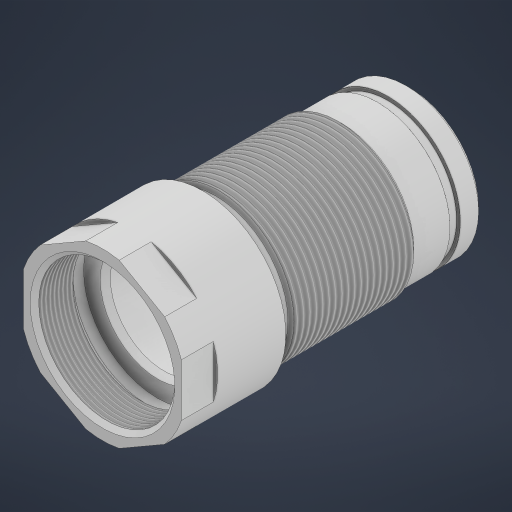
# Autodesk Inventor part: Переводник
Saved by Autodesk Inventor 2024.3 (Build 283343000, 343)
## iProperties
Created: 2025-08-06
Part Number: Переводник
Material: Generic
Document SubType Name: Modeling
Designer: LeoFB
Density: 1 g/cm^3
Appearance: Default
Author: LeoFB
Autodesk Inventor part; units mm, degrees
ref_plane "YZ Plane" through (0, 0, 0) normal (1, 0, 0) x (0, 1, 0)
ref_plane "XZ Plane" through (0, 0, 0) normal (0, 1, 0) x (-1, 0, 0)
ref_plane "XY Plane" through (0, 0, 0) normal (0, 0, 1) x (1, 0, 0)
sketch "Sketch1" plane through (0, 0, 0) normal (0, 1, 0) x (-1, 0, 0)
  line L0 (34, 0) -> (64.4, 0) construction
  line L1 (34, 32) -> (36, 32) construction
  line L2 (34, 91) -> (34, 97)
  line L3 (34, 97) -> (34, 91)
  line L4 (34, 91) -> (35.4142, 89.5858)
  line L5 (35.4142, 89.5858) -> (35.4142, 89.5858)
  line L6 (35.4142, 89.5858) -> (35.4142, 33.4142)
  line L7 (34, 97) -> (39, 97)
  line L8 (34, 97) -> (39, 97) construction
  line L9 (39, 97) -> (39, 129)
  line L10 (39, 129) -> (36, 129)
  line L11 (36, 129) -> (36, 144)
  line L12 (33.9171, 144) -> (36, 144)
  line L13 (31.9171, 142) -> (31.9171, 125.958)
  line L14 (31.9171, 144) -> (47.9592, 144) construction
  line L15 (31.9171, 125.958) -> (34.7455, 123.1296)
  line L16 (31.9171, 125.958) -> (35.9171, 125.958) construction
  line L17 (34.7455, 123.1296) -> (34.7455, 118.1296)
  line L18 (34.7455, 118.1296) -> (26.9171, 118.1296)
  line L19 (26.9171, 118.1296) -> (25.1856, 115.1305)
  line L20 (26.9171, 118.1296) -> (30.3802, 118.1296) construction
  line L21 (25.1856, 42.2286) -> (28.1856, 37.0325)
  line L22 (25.1856, 42.2286) -> (31.1856, 42.2286) construction
  line L23 (28.1856, 37.0325) -> (28.1856, 1.6)
  line L24 (32.4, 0) -> (29.7856, 0)
  line L25 (28.1856, 1.6) -> (29.7856, 0)
  line L26 (34, 1.6) -> (32.4, 0)
  line L27 (33.9171, 144) -> (31.9171, 142)
  line L28 (33.9, 14.92) -> (32.5, 14.92)
  line L29 (32.4, 14.82) -> (32.4, 10.32)
  line L30 (32.5, 10.22) -> (33.9, 10.22)
  line L31 (34, 1.6) -> (34, 10.12)
  arc A0 (32.5, 14.92) -> (32.4, 14.82) centre (32.5, 14.82) ccw
  arc A1 (32.4, 10.32) -> (32.5, 10.22) centre (32.5, 10.32) ccw
  arc A2 (33.9, 14.92) -> (34, 15.02) centre (33.9, 15.02) ccw
  arc A3 (34, 10.12) -> (33.9, 10.22) centre (33.9, 10.12) ccw
  line L32 (34, 15.02) -> (34, 32)
  line L33 (34, 32) -> (35.4142, 33.4142)
  line L34 (25.1856, 115.1305) -> (25.1856, 42.2286)
  line L35 (0, -28.8) -> (0, 172.8001) projected
  point P0 (0, 0)
  point P1 (28.1856, 0)
  point P2 (32.4, 14.92)
  point P3 (32.4, 10.22)
  dimension "d2" = 32
  dimension "d4" = 2
  dimension "d8" = 65
  dimension "d12" = 5
  dimension "d14" = 32
  dimension "d16" = 90
  dimension "d18" = 90
  dimension "d22" = 90
  dimension "d23" = 4
  dimension "d24" = 45
  dimension "d25" = 5
  dimension "d26" = 135
  dimension "d28" = 120
  dimension "d30" = 6
  dimension "d31" = 60
  dimension "d32" = 150
  dimension "d33" = 1.6
  dimension "d34" = 1.6
  dimension "d35" = 1.6
  dimension "d36" = 1.6
  dimension "d37" = 2
  dimension "d38" = 2
  dimension "d39" = 4.7
  dimension "d41" = 90
  dimension "d42" = 0.1
  constraints: 70 end point, 9 point on line, 8 horizontal, 8 point on circle, 7 perpendicular, 7 tangent, 5 equal length, 4 centre point, 4 vertical, 3 equal radius, 1 collinear, 1 parallel
  measures "d2" distance of L0.start L1.start
  measures "d4" distance of L1.start L6.end
  measures "d8" distance of L1.start L2.end
  measures "d12" distance of L2.end L7.end
  measures "d14" distance of L8.end L9.end
  measures "d16" angle of L10 L9
  measures "d18" angle of L10 L11
  measures "d22" angle of L13 L14
  measures "d23" distance of L13.end L15.end
  measures "d24" angle of L15 L16
  measures "d25" distance of L15.end L17.end
  measures "d26" angle of L15 L17
  measures "d28" angle of L19 L20
  measures "d30" distance of L21.start L21.end
  measures "d31" angle of L21 L22
  measures "d32" angle of L21 L23
  measures "d33" distance of L23.end point (28.186, 0)
  measures "d34" distance of L24.end point (28.186, 0)
  measures "d35" distance of L26.start L0.start
  measures "d36" distance of L24.start L0.start
  measures "d37" distance of L12.start L14.start
  measures "d38" distance of L13.start L14.start
  measures "d39" distance of point (32.4, 14.92) point (32.4, 10.22)
  measures "d41" angle of L30 L29
  measures "d42" radius of A0
revolve "Revolution1" add sketch "Sketch1" angle 360 about axis through (0, 0, -10) along (0, 0, 1)
thread "Thread1" size "M72x3" class "6g" standard "ANSI Metric M Profile" full length
thread "Thread2" size "M64x2" class "6H" standard "ANSI Metric M Profile" full length
sketch "Sketch2" plane through (0, 0, 144) normal (0, 0, 1) x (1, 0, 0)
  line L0 (29.1771, -25.8785) -> (7.8229, -38.2074)
  line L1 (-7.8229, -38.2074) -> (-29.1771, -25.8785)
  line L2 (-37, -12.3288) -> (-37, 12.3288)
  line L3 (-29.1771, 25.8785) -> (-7.8229, 38.2074)
  line L4 (7.8229, 38.2074) -> (29.1771, 25.8785)
  line L5 (37, 12.3288) -> (37, -12.3288)
  arc A0 (29.1771, -25.8785) -> (37, -12.3288) centre (0, 0) ccw
  arc A1 (37, 12.3288) -> (29.1771, 25.8785) centre (0, 0) ccw
  arc A2 (7.8229, 38.2074) -> (-7.8229, 38.2074) centre (0, 0) ccw
  arc A3 (-29.1771, 25.8785) -> (-37, 12.3288) centre (0, 0) ccw
  arc A4 (-37, -12.3288) -> (-29.1771, -25.8785) centre (0, 0) ccw
  arc A5 (-7.8229, -38.2074) -> (7.8229, -38.2074) centre (0, 0) ccw
  circle A6 centre (0, 0) radius 36
  dimension "d48" = 74
  constraints: 12 end point, 12 point on circle, 7 centre point, 3 coincident, 7 other
  measures "d48" distance between parallel lines of L3 L0
extrude "Extrusion1" add sketch "Sketch2" against normal blind 47
equation "\"d34\" = d33"
equation "\"d35\" = d33"
equation "\"d36\" = d35"
equation "\"d38\" = d37"
body "Solid1"
